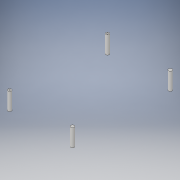
# Autodesk Inventor part: Trap
Saved by Autodesk Inventor 2019 (Build 230136000, 136)
## iProperties
Created: 2018-12-14
Part Number: Trap
Material: Generic
Document SubType Name: Modeling
Designer: jmc
Density: 1 g/cm^3
Appearance: Default
Author: jmc
Autodesk Inventor part; units mm, degrees
ref_plane "YZ Plane" through (0, 0, 0) normal (1, 0, 0) x (0, 1, 0)
ref_plane "XZ Plane" through (0, 0, 0) normal (0, 1, 0) x (-1, 0, 0)
ref_plane "Work Plane2" through (-20.1894, 38.7303, -132.5753) normal (0, -1, 0) x (1, 0, 0)
sketch "Sketch3" plane through (-20.2577, 38.7303, -13.8651) normal (0, -1, 0) x (0, 0, 1)
  circle A0 centre (-118.7102, -0.0683) radius 25 construction
  line L0 (-118.7102, -25.0683) -> (-118.7102, 24.9317) construction
  line L1 (0, 0) -> (-118.7102, -0.0683) construction
  circle A1 centre (71.2898, -90.0683) radius 2 projected
  circle A2 centre (-208.7102, -90.0683) radius 2 projected
  circle A3 centre (-208.7102, 89.9317) radius 2 projected
  circle A4 centre (71.2898, 89.9317) radius 2 projected
  circle A5 centre (71.2898, -90.0683) radius 5
  circle A6 centre (71.2898, 89.9317) radius 5
  circle A7 centre (-208.7102, -90.0683) radius 5
  circle A8 centre (-208.7102, 89.9317) radius 5
  dimension "d1" = 10
  dimension "d2" = 10
  dimension "d3" = 10
  dimension "d4" = 10
  constraints: 5 coincident, 4 centre point, 4 end point, 2 point on circle
  measures "d1" diameter of A5
  measures "d2" diameter of A6
  measures "d3" diameter of A7
  measures "d4" diameter of A8
extrude "Extrusion1" add sketch "Sketch3" along normal blind 50 contours A1 | A2 | A5 | A6 | A7 | A8
body "Solid1"
